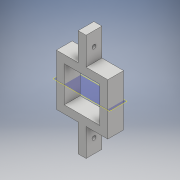
# Autodesk Inventor part: Support moteur pas a pas
Saved by Autodesk Inventor 2018 (Build 220112000, 112)
## iProperties
Created: 2018-05-14
Part Number: Support moteur pas a pas
Material: Générique
Document SubType Name: Modeling
Designer: Dimitri
Density: 1 g/cm^3
Appearance: Par défaut
Author: Dimitri
Autodesk Inventor part; units mm, degrees
ref_plane "YZ Plane" through (0, 0, 0) normal (1, 0, 0) x (0, 1, 0)
ref_plane "XZ Plane" through (0, 0, 0) normal (0, 1, 0) x (-1, 0, 0)
ref_plane "XY Plane" through (0, 0, 0) normal (0, 0, 1) x (1, 0, 0)
sketch "Esquisse1" plane through (0, 0, 0) normal (0, 1, 0) x (-1, 0, 0)
  line L0 (-22.5, 22.5) -> (22.5, 22.5)
  line L1 (22.5, 22.5) -> (22.5, -22.5)
  line L2 (22.5, -22.5) -> (-22.5, -22.5)
  line L3 (-22.5, -22.5) -> (-22.5, 22.5)
  line L4 (-22.5, 22.5) -> (22.5, -22.5) construction
  line L5 (22.5, 22.5) -> (-22.5, -22.5) construction
  line L6 (-32.5, 32.5) -> (32.5, 32.5)
  line L7 (32.5, 32.5) -> (32.5, -32.5)
  line L8 (32.5, -32.5) -> (-32.5, -32.5)
  line L9 (-32.5, -32.5) -> (-32.5, 32.5)
  line L10 (-32.5, 32.5) -> (32.5, -32.5) construction
  line L11 (32.5, 32.5) -> (-32.5, -32.5) construction
  point P0 (0, 0)
  dimension "d0" = 45
  dimension "d1" = 45
  dimension "d2" = 65
  constraints: 24 end point, 4 midpoint, 4 parallel, 2 horizontal, 2 perpendicular, 1 point on line
  measures "d0" distance of L1.end L2.end
  measures "d1" distance of L0.end L1.end
  measures "d2" distance of L7.end L8.end
extrude "Extrusion1" add sketch "Esquisse1" along normal blind 20
sketch "Esquisse2" plane through (-32.5, 0, 32.5) normal (0, 0, 1) x (1, 0, 0)
  line L0 (10, 20) -> (55, 20) projected
  line L1 (37.5, 0) -> (27.5, 0)
  line L2 (27.5, 0) -> (27.5, 20)
  line L3 (27.5, 20) -> (37.5, 20)
  line L4 (37.5, 20) -> (37.5, 0)
  line L5 (37.5, 0) -> (27.5, 20) construction
  line L6 (27.5, 0) -> (37.5, 20) construction
  point P0 (32.5, 0)
  dimension "d6" = 10
  constraints: 12 end point, 2 parallel, 1 horizontal, 1 perpendicular, 1 point on line
  measures "d6" distance of L2.end L3.end
extrude "Extrusion2" add sketch "Esquisse2" along normal blind 35
sketch "Esquisse3" plane through (5, 0, 32.5) normal (1, 0, 0) x (0, 0, -1)
  line L0 (-35, 0) -> (-35, 20) projected
  line L1 (0, 0) -> (0, 20) projected
  point P0 (32.5, 0)
  point P1 (-17.5, 10)
hole "Perçage1" at (5, 10, 50) direction (-1, 0, 0) diameter 5 end through all
mirror "Symétrie1" about plane through (0, 0, 0) normal (0, 0, 1) of "Extrusion2", "Perçage1"
ref_plane "Plan de construction1" through (0, 0, 0) normal (0, 0, 1) x (1, 0, 0)
